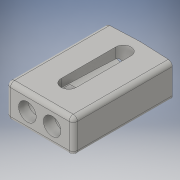
# Autodesk Inventor part: Part2
Saved by Autodesk Inventor 2016 (Build 200138000, 138)
## iProperties
Created: 2016-12-19
Part Number: Part2
Material: Generic
Document SubType Name: Modeling
Designer: Student
Density: 1 g/cm^3
Appearance: Default
Author: Student
Autodesk Inventor part; units mm, degrees
ref_plane "YZ Plane" through (0, 0, 0) normal (1, 0, 0) x (0, 1, 0)
ref_plane "XZ Plane" through (0, 0, 0) normal (0, 1, 0) x (-1, 0, 0)
ref_plane "XY Plane" through (0, 0, 0) normal (0, 0, 1) x (1, 0, 0)
sketch "Sketch1" plane through (6.985, -5.08, 0) normal (0, 0, 1) x (1, 0, 0)
  line L0 (-20.32, 10.16) -> (0, 10.16)
  line L1 (0, 10.16) -> (0, 0)
  line L2 (0, 0) -> (-20.32, 0)
  line L3 (-20.32, 0) -> (-20.32, 10.16)
  dimension "d0" = 20.32
  dimension "d1" = 10.16
  constraints: 8 end point, 2 parallel, 1 coincident, 1 horizontal, 1 perpendicular
  measures "d0" distance of L1.end L2.end
  measures "d1" distance of L0.end L1.end
extrude "Base Feature" add sketch "Sketch1" along normal blind 30.48
sketch "Sketch2" plane through (-13.335, -5.08, 0) normal (0, -1, 0) x (1, 0, 0)
  line L0 (0, 0) -> (20.32, 0) projected
  line L1 (10.16, 0) -> (20.32, 0.4436)
  line L2 (17.78, -1.2164) -> (10.16, -1.2164)
  line L3 (10.16, -1.2164) -> (10.16, 0)
  line L4 (10.16, 0) -> (0, 0.4436)
  line L5 (0, 0) -> (0, 30.48) projected
  line L6 (0, 0.4436) -> (0, -1.2164)
  line L7 (0, -1.2164) -> (20.32, -1.2164)
  line L8 (20.32, 0) -> (20.32, 30.48) projected
  line L9 (20.32, -1.2164) -> (20.32, 0.4436)
  dimension "d49" = 175
  dimension "d50" = 2.5
  dimension "d51" = 2.5
  constraints: 14 end point, 3 point on line, 2 midpoint, 2 perpendicular, 1 collinear, 1 vertical
  measures "d49" angle of L4 L1
  measures "d50" angle of L0 L1
  measures "d51" angle of L0 L4
extrude "Angled Cuts" cut sketch "Sketch2" against normal blind 25.4
sketch "Sketch4" plane through (6.985, -5.08, 0.4436) normal (0.0436194, 0, -0.9990482) x (-0.9990482, 0, -0.0436194)
  line L0 (0, 10.16) -> (10.1697, 10.16) projected
  line L1 (10.1697, 0) -> (0, 0) projected
  line L2 (10.1697, 0) -> (10.1697, 10.16) projected
  circle A0 centre (5.0848, 5.08) radius 3.175
  line L3 (0, 0) -> (0, 10.16) projected
  point P0 (6.9977, 5.08)
  dimension "d22" = 6.35
  dimension "d52" = 5.0848
  dimension "d53" = 5.08
  constraints: 1 centre point, 1 coincident
  measures "d22" diameter of A0
  measures "d52" distance from line of L2 point (5.085, 5.08)
  measures "d53" distance from line of L1 point (5.085, 5.08)
sketch "Sketch6" plane through (6.985, -5.08, 0.4436) normal (0.0436194, 0, -0.9990482) x (-0.9990482, 0, -0.0436194)
  circle A0 centre (5.0848, 5.08) radius 3.175 projected
  circle A1 centre (5.0848, 5.08) radius 2.667
  point P0 (6.9977, 5.08)
  dimension "d24" = 5.334
  constraints: 1 centre point, 1 coincident
  measures "d24" diameter of A1
sketch "Sketch7" plane through (-3.175, -5.08, 0) normal (-0.0436194, 0, -0.9990482) x (-0.9990482, 0, 0.0436194)
  circle A0 centre (5.0848, 5.08) radius 3.175
  circle A1 centre (5.0848, 5.08) radius 2.667
  line L0 (0, 10.16) -> (10.1697, 10.16) projected
  line L1 (0, 0) -> (0, 10.16)
  line L2 (10.1697, 0) -> (0, 0)
  line L3 (10.1697, 10.16) -> (10.1697, 0)
  dimension "d54" = 5.0848
  dimension "d55" = 5.08
  dimension "d56" = 5.334
  dimension "d60" = 6.35
  constraints: 6 end point, 2 centre point, 2 coincident
  measures "d54" distance from line of L3 point (5.085, 5.08)
  measures "d55" distance from line of L2 point (5.085, 5.08)
  measures "d56" diameter of A1
  measures "d60" diameter of A0
extrude "Extrusion4" cut sketch "Sketch4" against normal blind 27.178 contours A0
extrude "Extrusion5" cut sketch "Sketch7" against normal blind 27.178 contours A0
extrude "Extrusion6" cut sketch "Sketch6" against normal blind 50.8 contours A1
sketch "Sketch8" plane through (-8.255, 0, 0.2218) normal (-0.0436194, 0, -0.9990482) x (-0.9990482, 0, 0.0436194)
  circle A0 centre (0, 0) radius 2.667
  point P0 (-8.2568, 0)
  dimension "d34" = 5.334
  constraints: 1 centre point
  measures "d34" diameter of A0
extrude "Extrusion7" cut sketch "Sketch8" against normal blind 50.8
fillet "Fillet2" radius 1.27 8 edges at (-13.335, -5.08, 15.4618) (-13.335, 5.08, 15.4618) (6.985, -5.08, 15.4618) (6.985, 5.08, 15.4618) (-13.335, 0, 30.48) (6.985, 0, 30.48) (-3.175, -5.08, 30.48) (-3.175, 5.08, 30.48)
sketch "Sketch9" plane through (-12.065, 5.08, 29.21) normal (0, 1, 0) x (1, 0, 0)
  line L0 (0.0095, 28.6242) -> (8.8884, 28.9558) projected
  line L1 (8.89, 26.4321) -> (8.89, 5.1754) construction
  line L2 (6.5532, 24.0953) -> (6.5532, 7.5122)
  line L3 (11.2268, 7.5122) -> (11.2268, 24.0953)
  arc A0 (11.2268, 24.0953) -> (6.5532, 24.0953) centre (8.89, 24.0953) ccw
  arc A1 (6.5532, 7.5122) -> (11.2268, 7.5122) centre (8.89, 7.5122) ccw
  line L4 (6.3484, 27.1257) -> (27.6051, 27.1257) construction
  line L5 (0, 0) -> (0, 28.8219) projected
  point P0 (12.065, 29.21)
  point P1 (8.8884, 28.9558)
  point P2 (5.4296, 28.9214)
  point P3 (8.89, 15.8037)
  dimension "d45" = 90
  dimension "d46" = 4.6736
  dimension "d59" = 11.2268
  constraints: 10 end point, 6 point on circle, 4 tangent, 2 centre point, 2 point on line, 1 horizontal, 1 midpoint, 1 parallel, 1 perpendicular, 1 other
  measures "d45" angle of L1 L4
  measures "d46" diameter of A1
  measures "d59" distance between parallel lines of L5 L3
extrude "Extrusion8" cut sketch "Sketch9" against normal blind 50.8
sketch "Sketch10" plane through (6.985, -5.08, 30.48) normal (0, 0, 1) x (1, 0, 0)
  line L0 (-19.05, 8.89) -> (-1.27, 8.89) projected
  line L1 (-1.27, 1.27) -> (-19.05, 1.27) projected
  line L2 (-11.1828, 8.615) -> (-9.1508, 8.615)
  line L3 (-9.1508, 8.615) -> (-9.1508, 1.5266)
  line L4 (-9.1508, 1.5266) -> (-11.1828, 1.5266)
  line L5 (-11.1828, 1.5266) -> (-11.1828, 8.615)
  point P0 (-6.985, 5.08)
  dimension "d61" = 2.032
  constraints: 8 end point, 2 parallel, 1 horizontal, 1 perpendicular
  measures "d61" distance between parallel lines of L5 L3
extrude "Extrusion9" add sketch "Sketch10" against normal blind 10.16
body "Solid1"
